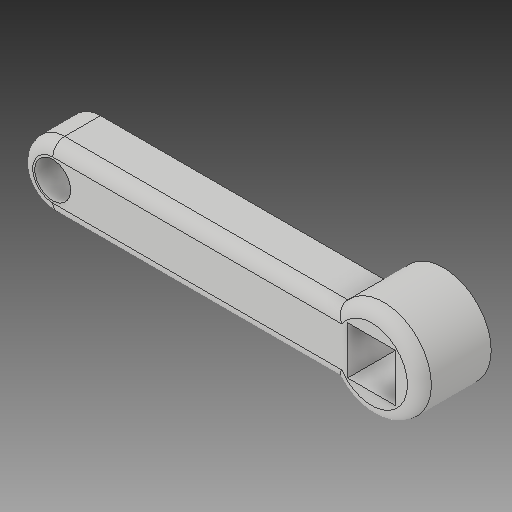
# Autodesk Inventor part: crankshaft
Saved by Autodesk Inventor 2017 (Build 210142000, 142)
## iProperties
Created: 2020-03-22
Part Number: crankshaft
Material: Generic
Document SubType Name: Modeling
Designer: LaNave
Density: 1 g/cm^3
Appearance: Default
Mass: 1.13433 g
Surface Area: 12.335 cm^2
Volume: 1.13433 cm^3
Author: LaNave
Autodesk Inventor part; units mm, degrees
ref_plane "YZ Plane" through (0, 0, 0) normal (1, 0, 0) x (0, 1, 0)
ref_plane "XZ Plane" through (0, 0, 0) normal (0, 1, 0) x (-1, 0, 0)
ref_plane "XY Plane" through (0, 0, 0) normal (0, 0, 1) x (1, 0, 0)
sketch "Sketch1" plane through (0, 0, 0) normal (0, 0, 1) x (1, 0, 0)
  circle A0 centre (-39.9943, 0) radius 2.25
  arc A1 (-5.0436, -3.25) -> (-5.0436, 3.25) centre (0, 0) ccw
  line L0 (3, 3) -> (3, -3)
  line L1 (3, -3) -> (-3, -3)
  line L2 (-3, -3) -> (-3, 3)
  line L3 (-3, 3) -> (3, 3)
  line L4 (-3, 3) -> (3, 3)
  line L5 (-3, -3) -> (3, -3)
  line L6 (-39.9943, -4) -> (-4.4721, -4)
  line L7 (-4.4721, 4) -> (-39.9943, 4)
  arc A2 (-39.9943, 4) -> (-39.9943, -4) centre (-39.9943, 0) ccw
  point P0 (0, 3)
  point P1 (-19.9972, 0)
  constraints: 16 end point, 6 point on circle, 3 centre point, 2 horizontal, 2 midpoint, 2 tangent, 1 coincident, 1 parallel
extrude "Extrusion1" add sketch "Sketch1" along normal blind 6
sketch "Sketch5" plane through (0, 0, 0) normal (0, 0, -1) x (-1, 0, 0)
  circle A0 centre (0, 0) radius 6
  arc A1 (4.4721, 4) -> (4.4721, -4) centre (0, 0) ccw projected
  line L0 (-3, -3) -> (-3, 3)
  line L1 (-3, 3) -> (3, 3)
  line L2 (3, 3) -> (3, -3)
  line L3 (3, -3) -> (-3, -3)
  point P0 (2.804, -2.804)
  point P1 (5.0436, -3.25)
  point P2 (5.0436, 3.25)
  point P3 (0, -3)
  constraints: 8 end point, 2 coincident, 1 centre point, 1 midpoint, 9 other
extrude "Extrusion5" add sketch "Sketch5" along normal blind 3
fillet "Fillet2" radius 1.5 4 edges at (-22.2332, -4, 6) (-43.9943, 0, 6) (-22.2332, 4, 6) (6, 0, 6)
scale "Scale1" factors (0.5, 0.5, 0.5) then translate (-11.1166, 2, 0) bodies 1
body "Solid1"
